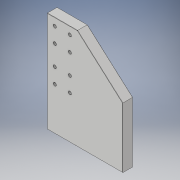
# Autodesk Inventor part: Portalwange
Saved by Autodesk Inventor 2019 (Build 230136000, 136)
## iProperties
Created: 2021-05-10
Part Number: Portalwange
Material: Generic
Document SubType Name: Modeling
Designer: Lenovo
Density: 1 g/cm^3
Appearance: Default
Author: Lenovo
Autodesk Inventor part; units mm, degrees
ref_plane "YZ Plane" through (0, 0, 0) normal (1, 0, 0) x (0, 1, 0)
ref_plane "XZ Plane" through (0, 0, 0) normal (0, 1, 0) x (-1, 0, 0)
ref_plane "XY Plane" through (0, 0, 0) normal (0, 0, 1) x (1, 0, 0)
sketch "Skizze1" plane through (0, 0, 0) normal (0, 0, 1) x (1, 0, 0)
  line L0 (0, 0) -> (0, 200)
  line L1 (0, 200) -> (60, 200)
  line L2 (0, 0) -> (150, 0)
  line L3 (150, 0) -> (150, 120)
  line L4 (150, 120) -> (60, 200)
  dimension "d0" = 200
  dimension "d1" = 60
  dimension "d2" = 150
  dimension "d3" = 120
  constraints: 10 end point, 2 perpendicular, 1 horizontal, 1 vertical
  measures "d0" distance of L0.start L0.end
  measures "d1" distance of L0.end L1.end
  measures "d2" distance of L0.start L2.end
  measures "d3" distance of L2.end L3.end
extrude "Extrusion1" add sketch "Skizze1" along normal blind 20
sketch "Skizze2" plane through (0, 0, 20) normal (0, 0, 1) x (1, 0, 0)
  line L0 (60, 200) -> (0, 200) projected
  line L1 (30, 200) -> (30, 170) construction
  line L2 (30, 170) -> (30, 100) construction
  line L3 (15, 155) -> (45, 155) construction
  line L4 (45, 155) -> (45, 185) construction
  line L5 (45, 185) -> (15, 185) construction
  line L6 (15, 185) -> (15, 155) construction
  line L7 (15, 155) -> (45, 185) construction
  line L8 (45, 155) -> (15, 185) construction
  line L9 (15, 85) -> (45, 85) construction
  line L10 (45, 85) -> (45, 115) construction
  line L11 (45, 115) -> (15, 115) construction
  line L12 (15, 115) -> (15, 85) construction
  line L13 (15, 85) -> (45, 115) construction
  line L14 (45, 85) -> (15, 115) construction
  point P0 (0, 0)
  dimension "d6" = 30
  dimension "d7" = 70
  dimension "d8" = 30
  dimension "d9" = 30
  dimension "d10" = 30
  dimension "d11" = 30
  constraints: 28 end point, 5 midpoint, 4 parallel, 2 horizontal, 2 perpendicular, 1 point on line, 1 vertical
  measures "d6" distance of L1.start L1.end
  measures "d7" distance of L1.end L2.end
  measures "d8" distance of L5.end L4.end
  measures "d9" distance of L4.end L3.end
  measures "d10" distance of L11.end L10.end
  measures "d11" distance of L10.end L9.end
hole "Bohrung1" at (15, 185, 20) at (45, 185, 20) at (15, 155, 20) at (45, 155, 20) at (15, 115, 20) at (45, 115, 20) at (15, 85, 20) at (45, 85, 20) direction (0, 0, -1) diameter 5.5 end through all clearance for "Sechskantkopfschraube ISO 24017" size "M5" standard "ISO"
chamfer "Fase1" distance 0.5 angle 45 18 edges at (30, 200, 20) (105, 160, 20) (150, 60, 20) (75, 0, 20) (0, 100, 20) (15, 117.75, 20) (45, 117.75, 20) (45, 87.75, 20) (15, 87.75, 20) (15, 157.75, 20) (45, 157.75, 20) (15, 187.75, 20) (45, 187.75, 20) (105, 160, 0) (30, 200, 0) (0, 100, 0) (150, 60, 0) (75, 0, 0)
chamfer "Fase2" distance 0.5 angle 45 8 edges at (15, 187.75, 0) (15, 157.75, 0) (15, 117.75, 0) (15, 87.75, 0) (45, 87.75, 0) (45, 117.75, 0) (45, 157.75, 0) (45, 187.75, 0)
